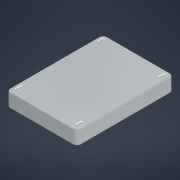
# Autodesk Inventor part: box
Saved by Autodesk Inventor 2021 (Build 250183000, 183)
## iProperties
Created: 2023-03-30
Part Number: box
Material: ガラス
Document SubType Name: Modeling
Designer: casey
Density: 2.18 g/cm^3
Appearance: クリア
Author: casey
Autodesk Inventor part; units mm, degrees
ref_plane "YZ Plane" through (0, 0, 0) normal (1, 0, 0) x (0, 1, 0)
ref_plane "XZ Plane" through (0, 0, 0) normal (0, 1, 0) x (-1, 0, 0)
ref_plane "XY Plane" through (0, 0, 0) normal (0, 0, 1) x (1, 0, 0)
sketch "スケッチ2" plane through (0, 0, 0) normal (0, 1, 0) x (-1, 0, 0)
  line L0 (0, 0) -> (-170, 0)
  line L1 (-170, 0) -> (-170, -233)
  line L2 (-170, -233) -> (0, -233)
  line L3 (0, -233) -> (0, 0)
  dimension "d0" = 170
  dimension "d1" = 233
  constraints: 8 end point, 2 parallel, 1 horizontal, 1 perpendicular
  measures "d0" distance of L2.end L1.end
  measures "d1" distance of L1.end L0.end
extrude "押し出し1" add sketch "スケッチ2" along normal blind 34
fillet "フィレット1" radius 10 4 edges at (170, 17, 0) (0, 17, 0) (170, 17, -233) (0, 17, -233)
fillet "フィレット2" radius 3 16 edges at (167.0711, 34, -2.9289) (170, 34, -116.5) (167.0711, 34, -230.0711) (85, 34, -233) (2.9289, 34, -230.0711) (0, 34, -116.5) (2.9289, 34, -2.9289) (85, 34, 0) (167.0711, 0, -230.0711) (85, 0, -233) (2.9289, 0, -230.0711) (0, 0, -116.5) (2.9289, 0, -2.9289) (85, 0, 0) (167.0711, 0, -2.9289) (170, 0, -116.5)
sketch "スケッチ3" plane through (0, 34, 0) normal (0, 1, 0) x (1, 0, 0)
  line L0 (10, 10) -> (13, 10)
  line L1 (13, 10) -> (13, 25)
  line L2 (13, 25) -> (10, 25)
  line L3 (10, 25) -> (10, 10)
  line L4 (0, 223) -> (0, 10) projected
  line L5 (10, 0) -> (160, 0) projected
  line L6 (157, 10) -> (160, 10)
  line L7 (160, 10) -> (160, 25)
  line L8 (160, 25) -> (157, 25)
  line L9 (157, 25) -> (157, 10)
  line L10 (170, 10) -> (170, 223) projected
  arc A0 (170, 223) -> (160, 233) centre (160, 223) ccw projected
  line L11 (160, 223) -> (157, 223)
  line L12 (157, 223) -> (157, 208)
  line L13 (157, 208) -> (160, 208)
  line L14 (160, 208) -> (160, 223)
  arc A1 (10, 233) -> (0, 223) centre (10, 223) ccw projected
  line L15 (10, 223) -> (13, 223)
  line L16 (13, 223) -> (13, 208)
  line L17 (13, 208) -> (10, 208)
  line L18 (10, 208) -> (10, 223)
  point P0 (0, 0)
  dimension "d6" = 3
  dimension "d7" = 15
  dimension "d8" = 10
  dimension "d9" = 10
  dimension "d10" = 3
  dimension "d11" = 15
  dimension "d12" = 10
  dimension "d13" = 10
  dimension "d14" = 3
  dimension "d15" = 15
  dimension "d16" = 3
  dimension "d17" = 15
  constraints: 32 end point, 8 parallel, 4 horizontal, 4 perpendicular
  measures "d6" distance of L2.end L1.end
  measures "d7" distance of L1.end L0.end
  measures "d8" distance between parallel lines of L4 L3
  measures "d9" distance between parallel lines of L5 L0
  measures "d10" distance of L8.end L7.end
  measures "d11" distance of L7.end L6.end
  measures "d12" distance from line of L5 L6.end
  measures "d13" distance between parallel lines of L10 L7
  measures "d14" distance of L13.end L12.end
  measures "d15" distance of L12.end L11.end
  measures "d16" distance of L16.end L17.end
  measures "d17" distance of L15.end L16.end
extrude "押し出し2" add sketch "スケッチ3" along normal blind 3
